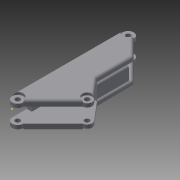
# Autodesk Inventor part: Finger_Lower_main_1
Saved by Autodesk Inventor 2015 (Build 190159000, 159)
## iProperties
Created: 2016-07-06
Part Number: Finger_Lower_main_1
Material: Generic
Document SubType Name: Modeling
Designer: Neelotpal Nag
Density: 1 g/cm^3
Appearance: Default
Author: Neelotpal Nag
Autodesk Inventor part; units mm, degrees
ref_plane "YZ Plane" through (0, 0, 0) normal (1, 0, 0) x (0, 1, 0)
ref_plane "XZ Plane" through (0, 0, 0) normal (0, 1, 0) x (-1, 0, 0)
sketch "Sketch1" plane through (0, 0, 0) normal (0, 0, 1) x (1, 0, 0)
  line L0 (0, 0) -> (0, 45)
  line L1 (0, 0) -> (14.1421, 14.1421)
  line L2 (0, 0) -> (20, 0) construction
  line L3 (14.1421, 14.1421) -> (0, 14.1421)
  circle A0 centre (0, 0) radius 1
  circle A1 centre (14.1421, 14.1421) radius 1
  circle A2 centre (0, 45) radius 1
  circle A3 centre (0, 0) radius 2.25
  circle A4 centre (0, 45) radius 2.25
  dimension "d0" = 45
  dimension "d1" = 20
  dimension "d2" = 45
  dimension "d3" = 2
  dimension "d4" = 2
  dimension "d5" = 2
  dimension "d6" = 4.5
  dimension "d10" = 4.5
  constraints: 8 coincident, 8 end point, 5 centre point, 1 equal length, 1 horizontal, 1 perpendicular, 1 point on line, 1 vertical
  measures "d0" distance of L0.start L0.end
  measures "d1" distance of L1.start L1.end
  measures "d2" angle of L2 L1
  measures "d3" diameter of A0
  measures "d4" diameter of A1
  measures "d5" diameter of A2
  measures "d6" diameter of A3
  measures "d10" diameter of A4
ref_plane "Work Plane1" through (0, 0, 3) normal (0, 0, 1) x (1, 0, 0)
sketch "Sketch2" plane through (0, 0, 3) normal (0, 0, 1) x (1, 0, 0)
  circle A0 centre (0, 0) radius 1 projected
  circle A1 centre (0, 0) radius 2.25 projected
  circle A2 centre (14.1421, 14.1421) radius 1 projected
  circle A3 centre (0, 45) radius 1 projected
  circle A4 centre (0, 45) radius 2.25 projected
  line L0 (0, 0) -> (0, 45) projected
extrude "Extrusion1" add sketch "Sketch2" along normal blind 1.5 contours A1
sketch "Sketch3" plane through (0, 0, 3) normal (0, 0, 1) x (1, 0, 0)
  point P0 (0, 0)
extrude "Extrusion2" add sketch "Sketch2" along normal blind 1.5 contours A4
sketch "Sketch4" plane through (0, 0, 3) normal (0, 0, 1) x (1, 0, 0)
  circle A0 centre (0, 0) radius 2.25 projected
  line L0 (-2.25, 0) -> (-2.25, 45)
  circle A1 centre (0, 45) radius 2.25 projected
  line L1 (2.25, 45) -> (9.3211, 37.9289)
  line L2 (2.25, 45) -> (12.25, 45) construction
  line L3 (9.3211, 37.9289) -> (9.3211, 22.9289)
  dimension "d13" = 10
  dimension "d14" = 45
  dimension "d15" = 15
  constraints: 8 end point, 2 point on circle, 1 equal length, 1 horizontal, 1 horizontal alignment, 1 parallel, 1 tangent, 1 vertical, 1 other
  measures "d13" distance of L1.start L1.end
  measures "d14" angle of L1 L2
  measures "d15" distance of L1.end L3.end
sketch "Sketch5" plane through (0, 0, 3) normal (0, 0, 1) x (1, 0, 0)
  circle A0 centre (14.1421, 14.1421) radius 1 projected
  circle A1 centre (14.1421, 14.1421) radius 2
  point P0 (0, 0)
  dimension "d16" = 4
  constraints: 1 centre point, 1 coincident
  measures "d16" diameter of A1
extrude "Extrusion3" add sketch "Sketch5" along normal blind 1.5
sketch "Sketch6" plane through (0, 0, 3) normal (0, 0, 1) x (1, 0, 0)
  circle A0 centre (0, 45) radius 2.25 projected
  line L0 (2.25, 45) -> (9.3211, 37.9289)
  line L1 (2.25, 45) -> (12.25, 45) construction
  line L2 (9.3211, 37.9289) -> (9.3211, 22.9289)
  line L3 (9.3211, 22.9289) -> (15.6683, 15.4347)
  circle A1 centre (14.1421, 14.1421) radius 2 projected
  line L4 (-2.25, 45) -> (-2.25, 0)
  circle A2 centre (0, 0) radius 2.25 projected
  circle A3 centre (14.1421, 14.1421) radius 2 projected
  circle A4 centre (14.1421, 14.1421) radius 1 projected
  line L5 (2.25, 0) -> (14.4102, 12.1602)
  line L6 (2.25, 0) -> (19.4471, 0) construction
  arc A5 (-2.25, 45) -> (2.25, 45) centre (0, 45) ccw
  line L7 (2.25, 45) -> (9.3211, 37.9289)
  line L8 (9.3211, 22.9289) -> (9.3211, 37.9289)
  line L9 (9.3211, 22.9289) -> (15.6683, 15.4347)
  line L10 (14.4102, 12.1602) -> (2.25, 0)
  circle A6 centre (14.1421, 14.1421) radius 2
  circle A7 centre (0, 0) radius 2.25
  line L11 (-2.25, 0) -> (-2.25, 45)
  circle A8 centre (0, 45) radius 2.25
  arc A9 (-2.25, 45) -> (2.25, 45) centre (0, 45) ccw
  arc A10 (15.6683, 15.4347) -> (14.4102, 12.1602) centre (14.1421, 14.1421) ccw
  arc A11 (2.25, 0) -> (-2.25, 0) centre (0, 0) ccw
  dimension "d19" = 10
  dimension "d20" = 45
  dimension "d21" = 15
  dimension "d22" = 45
  constraints: 24 end point, 12 point on circle, 7 centre point, 7 tangent, 6 concentric, 3 coincident, 3 collinear, 2 equal length, 2 horizontal, 1 vertical, 7 other
  measures "d19" distance of L0.start L0.end
  measures "d20" angle of L0 L1
  measures "d21" distance of L0.end L2.end
  measures "d22" angle of L6 L5
extrude "Extrusion4" add sketch "Sketch6" along normal blind 2.5 contours L0 L2 L3 A1 L5 A2 L4 A0
fillet "Fillet1" radius 1 1 edges at (9.3211, 30.4289, 5.5)
fillet "Fillet2" radius 1 1 edges at (9.3211, 30.4289, 3)
fillet "Fillet3" radius 1 5 edges at (5.2855, 41.9645, 5.5) (9.0282, 38.2218, 5.2071) (9.3211, 37.9289, 4.25) (9.0282, 38.2218, 3.2929) (5.2855, 41.9645, 3)
fillet "Fillet4" radius 1 1 edges at (11.9947, 19.7722, 5.5)
fillet "Fillet5" radius 1 1 edges at (8.3301, 6.0801, 5.5)
fillet "Fillet6" radius 1 1 edges at (-2.25, 22.5, 5.5)
mirror "Mirror1" about plane through (0, 0, 0) normal (0, 0, 1) of "Extrusion4"
mirror "Mirror2" about plane through (0, 0, 0) normal (0, 0, 1) of "Extrusion2", "Extrusion3", "Extrusion1"
sketch "Sketch7" plane through (-2.25, 0, -5.5) normal (-1, 0, 0) x (0, 0, 1)
  point P0 (5.5, 0)
sketch "Sketch8" plane through (-2.25, 0, -5.5) normal (-1, 0, 0) x (0, 0, 1)
  line L0 (2.5, 45) -> (2.5, 0) projected
  line L1 (8.5, 45) -> (8.5, 0) projected
  line L2 (2.5, 6) -> (8.5, 6)
  line L3 (8.5, 6) -> (8.5, 36)
  line L4 (8.5, 36) -> (2.5, 36)
  line L5 (2.5, 36) -> (2.5, 6)
  point P0 (5.5, 0)
  dimension "d31" = 30
  constraints: 8 end point, 2 parallel, 2 point on line, 1 horizontal, 1 perpendicular
  measures "d31" distance of L3.end L2.end
extrude "Extrusion5" add sketch "Sketch8" against normal blind 2
fillet "Fillet7" radius 1 1 edges at (9.3211, 30.4289, -5.5)
fillet "Fillet8" radius 1 2 edges at (8.8211, 23.5193, -5.5) (12.4947, 19.1818, -5.5)
fillet "Fillet9" radius 1 1 edges at (8.3301, 6.0801, -5.5)
fillet "Fillet10" radius 1 1 edges at (-2.25, 22.5, -5.5)
fillet "Fillet11" radius 1 3 edges at (5.2855, 41.9645, -5.5) (9.0282, 38.2218, -5.2071) (9.3211, 37.9289, -3.75)
sketch "Sketch9" plane through (9.3211, 22.9289, -3) normal (1, 0, 0) x (0, 0, -1)
  line L0 (-6, 13.0711) -> (0, 13.0711)
  line L1 (0, 13.0711) -> (0, 0)
  line L2 (0, 0) -> (-6, 0)
  line L3 (-6, 0) -> (-6, 13.0711)
  point P0 (-3, -22.9289)
  constraints: 8 end point, 2 parallel, 1 horizontal, 1 perpendicular
fillet "Fillet12" radius 1 3 edges at (9.2449, 37.8974, -3) (5.6391, 41.6109, -3) (9.3211, 30.2218, -3)
extrude "Extrusion6" add sketch "Sketch9" against normal blind 2
fillet "Fillet13" radius 1 1 edges at (9.3211, 29.4645, 3)
fillet "Fillet14" radius 1 1 edges at (9.3211, 29.4645, -3)
sketch "Sketch10" plane through (-2.25, 0, 4.5) normal (-1, 0, 0) x (0, 0, 1)
  line L0 (-4.5, 0) -> (-4.5, 35.7983)
  line L1 (-7.5, 6) -> (-1.5, 6) projected
  line L2 (-6.5, 22.9289) -> (-2.5, 22.9289) projected
  line L3 (-5.5, 6.4068) -> (-3.5, 6.4068)
  line L4 (-3.5, 6.4068) -> (-3.5, 26.4068)
  line L5 (-3.5, 26.4068) -> (-5.5, 26.4068)
  line L6 (-5.5, 26.4068) -> (-5.5, 6.4068)
  line L7 (-5.5, 6.4068) -> (-3.5, 26.4068) construction
  line L8 (-3.5, 6.4068) -> (-5.5, 26.4068) construction
  line L9 (-5.5, 26.4068) -> (-5.5407, 6)
  line L10 (-3.5, 26.4068) -> (-3.5, 6)
  line L11 (-5.5407, 6) -> (-3.5, 6)
  point P0 (-4.5, 6)
  point P1 (-4.5, 22.9289)
  point P2 (-4.5, 16.4068)
  dimension "d44" = 2
  dimension "d45" = 20
  constraints: 20 end point, 5 point on line, 4 midpoint, 2 parallel, 1 coincident, 1 collinear, 1 horizontal, 1 perpendicular, 1 vertical
  measures "d44" distance of L5.end L4.end
  measures "d45" distance of L4.end L3.end
extrude "Extrusion7" cut sketch "Sketch10" against normal blind 2
ref_plane "Work Plane2" through (0, 0, 0) normal (0, 0, 1) x (1, 0, 0)
body "Solid1"
